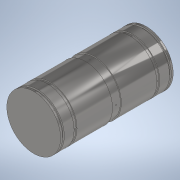
# Autodesk Inventor part: Палец
Saved by Autodesk Inventor 2021 (Build 250183000, 183)
## iProperties
Created: 2020-11-30
Part Number: Палец
Material: Сталь, высокопрочная, низколегированная
Document SubType Name: Modeling
Designer: Тимоха
Mass: 14180.4 g
Surface Area: 879.646 cm^2
Volume: 1806.42 cm^3
Density: 7.85 g/cm^3
Appearance: Сталь — полированная
Author: Тимоха
Autodesk Inventor part; units mm, degrees
ref_plane "YZ Plane" through (0, 0, 0) normal (1, 0, 0) x (0, 1, 0)
ref_plane "XZ Plane" through (0, 0, 0) normal (0, 1, 0) x (-1, 0, 0)
ref_plane "XY Plane" through (0, 0, 0) normal (0, 0, 1) x (1, 0, 0)
sketch "Эскиз1" plane through (0, 0, 0) normal (0, 0, 1) x (1, 0, 0)
  circle A0 centre (0, 0) radius 55
  dimension "d0" = 110
  constraints: 1 centre point, 1 coincident
  measures "d0" diameter of A0
extrude "Выдавливание1" add sketch "Эскиз1" along normal blind 230
sketch "Эскиз2" plane through (0, 0, 0) normal (0, 1, 0) x (-1, 0, 0)
  line L0 (55, 0) -> (-55, 0) projected
  line L1 (-55, 0) -> (-55, 230) projected
  line L2 (55, 230) -> (-55, 230) projected
  line L3 (-55, 230) -> (-55, 222.5)
  line L4 (-55, 222.5) -> (-52, 222.5)
  line L5 (-52, 222.5) -> (-52, 226)
  line L6 (-52, 226) -> (-55, 226)
  line L7 (0, -46) -> (0, 276) projected
  line L8 (-55, 0) -> (-55, 7.5)
  line L9 (-55, 0) -> (-55, 230) projected
  line L10 (-55, 7.5) -> (-52, 7.5)
  line L11 (-52, 7.5) -> (-52, 4)
  line L12 (-52, 4) -> (-55, 4)
  line L13 (-55, 0) -> (-55, 230) projected
  line L14 (-55, 7.5) -> (-55, 27.5)
  line L15 (-55, 0) -> (-55, 230) projected
  line L16 (-55, 27.5) -> (-53, 27.5)
  line L17 (-53, 27.5) -> (-53, 33.5)
  line L18 (-53, 33.5) -> (-55, 33.5)
  line L19 (-55, 0) -> (-55, 230) projected
  line L20 (-55, 222.5) -> (-55, 202.5)
  line L21 (-55, 0) -> (-55, 230) projected
  line L22 (-55, 202.5) -> (-53, 202.5)
  line L23 (-53, 202.5) -> (-53, 196.5)
  line L24 (-53, 196.5) -> (-55, 196.5)
  line L25 (-55, 0) -> (-55, 230) projected
  line L26 (-55, 0) -> (-55, 230) projected
  line L27 (-55, 55) -> (-55, 106)
  line L28 (-55, 0) -> (-55, 230) projected
  line L29 (-55, 106) -> (-53, 106)
  line L30 (-53, 106) -> (-53, 124)
  line L31 (-53, 124) -> (-55, 124)
  line L32 (-55, 0) -> (-55, 230) projected
  point P0 (0, 0)
  dimension "d3" = 7.5
  dimension "d5" = 7.5
  dimension "d6" = 3.5
  dimension "d7" = 20
  dimension "d8" = 2
  dimension "d9" = 6
  dimension "d10" = 20
  dimension "d11" = 2
  dimension "d12" = 6
  dimension "d13" = 51
  dimension "d14" = 18
  constraints: 40 end point, 12 perpendicular, 5 point on line, 2 horizontal, 17 other
  measures "d3" distance of L2.end L3.end
  measures "d5" distance of L8.start L8.end
  measures "d6" distance of L10.end L11.end
  measures "d7" distance of L8.end L14.end
  measures "d8" distance of L14.end L16.end
  measures "d9" distance of L16.end L17.end
  measures "d10" distance of L3.end L20.end
  measures "d11" distance of L20.end L22.end
  measures "d12" distance of L22.end L23.end
  measures "d13" distance of L27.start L27.end
  measures "d14" distance of L29.end L30.end
revolve "Вращение1" cut sketch "Эскиз2" angle 360 about axis through (0, 0, -10) along (0, 0, 1) contours L1 L10 L11 L12 | L6 L5 L4 L1 | L1 L18 L17 L16 | L22 L23 L24 L1 | L1 L31 L30 L29
sketch "Эскиз3" plane through (0, 0, 0) normal (1, 0, 0) x (0, 1, 0)
  line L0 (-53, 27.5) -> (-53, 33.5) projected
  line L1 (-53, 33.5) -> (53, 33.5) projected
  line L2 (55, 33.5) -> (-55, 33.5) projected
  line L3 (0, 33.5) -> (0, 30.5)
  circle A0 centre (0, 30.5) radius 1
  line L4 (-53, 106) -> (53, 106) projected
  line L5 (0, 106) -> (0, 115)
  circle A1 centre (0, 115) radius 1
  line L6 (-53, 196.5) -> (53, 196.5) projected
  line L7 (0, 196.5) -> (0, 199.5)
  circle A2 centre (0, 199.5) radius 1
  point P0 (0, 0)
  dimension "d15" = 2
  dimension "d16" = 3
  constraints: 6 end point, 3 centre point, 3 coincident, 3 midpoint, 3 vertical
  measures "d15" diameter of A1
  measures "d16" distance of L7.start L7.end
extrude "Выдавливание2" cut sketch "Эскиз3" against normal through all both and the other way through all
sketch "Эскиз4" plane through (0, 0, 0) normal (0, 1, 0) x (-1, 0, 0)
  line L0 (-53, 29.5) -> (53, 29.5) projected
  line L1 (0, 29.5) -> (0, 30.5)
  circle A0 centre (0, 30.5) radius 1
  line L2 (-53, 114) -> (53, 114) projected
  line L3 (0, 114) -> (0, 115)
  circle A1 centre (0, 115) radius 1
  line L4 (-53, 198.5) -> (53, 198.5) projected
  line L5 (0, 198.5) -> (0, 199.5)
  circle A2 centre (0, 199.5) radius 1
  point P0 (0, 0)
  dimension "d19" = 1
  dimension "d20" = 1
  constraints: 6 end point, 3 coincident, 3 midpoint, 3 vertical, 3 vertical alignment, 6 other
  measures "d19" distance of L1.start L1.end
  measures "d20" distance of L5.start L5.end
extrude "Выдавливание3" cut sketch "Эскиз4" against normal through all both and the other way through all
